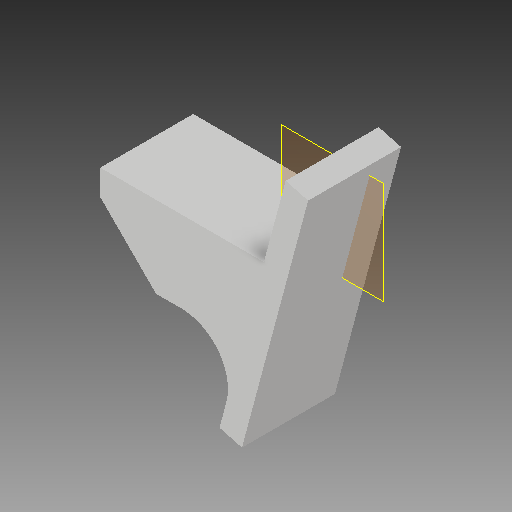
# Autodesk Inventor part: Stand_Back
Saved by Autodesk Inventor 2018 (Build 220112000, 112)
## iProperties
Created: 2018-02-04
Part Number: Stand_Back
Material: Generic
Document SubType Name: Modeling
Designer: Mandus
Density: 1 g/cm^3
Appearance: Default
Author: Mandus
Autodesk Inventor part; units mm, degrees
ref_plane "YZ Plane" through (0, 0, 0) normal (1, 0, 0) x (0, 1, 0)
sketch "Sketch1" plane through (0, 0, 0) normal (0, 0, 1) x (1, 0, 0)
  line L0 (36, 0.51) -> (25.6472, -38.1271)
  line L1 (36, 0.51) -> (76, 0.51) construction
  line L2 (36, 0.51) -> (25.6472, -38.1271) construction
  line L3 (25.6472, -38.1271) -> (30.4769, -39.4212)
  line L4 (30.4769, -39.4212) -> (40.8296, -0.7841)
  line L5 (40.8296, -0.7841) -> (36, 0.51)
  line L6 (36, 0.51) -> (40.8296, -0.7841)
  line L7 (40.8296, -0.7841) -> (44.7119, 13.7048)
  line L8 (44.7119, 13.7048) -> (39.8823, 14.9989)
  line L9 (39.8823, 14.9989) -> (36, 0.51)
  arc A0 (36, -1.5) -> (26, 8.5) centre (26, -1.5) ccw construction
  line L10 (39.0787, 12) -> (34.0787, 12)
  line L11 (34.0787, 12) -> (34.0787, 9)
  line L12 (34.0787, 9) -> (38.2749, 9)
  line L13 (14, -12.5) -> (26, -12.5) construction
  line L14 (0, -20) -> (30.5044, -20)
  line L15 (30.5044, -20) -> (35.8634, 0)
  line L16 (35.1935, -2.5) -> (0, -2.5)
  line L17 (35.1935, -2.5) -> (30.5044, -20)
  line L18 (0, -20) -> (0, -2.5)
  line L19 (-41.5, -2.5) -> (36, -2.5) construction
  line L20 (30.5044, -20) -> (35.1935, -2.5) construction
  point P0 (0, 0)
  point P1 (17.5967, -2.5)
  dimension "d0" = 40
  dimension "d1" = 105
  dimension "d2" = 5
  dimension "d3" = 15
  dimension "d5" = 5
  dimension "d6" = 3
  dimension "d7" = 11.49
  dimension "d20" = 17.5
  dimension "d21" = 35.1935
  dimension "d22" = 30.5044
  constraints: 42 end point, 5 point on line, 4 collinear, 4 horizontal, 4 parallel, 3 perpendicular, 3 vertical, 1 equal length, 1 horizontal alignment, 1 midpoint, 4 other
  measures "d0" distance of L0.start L0.end
  measures "d1" angle of L0 L1
  measures "d2" distance of L3.end L0.end
  measures "d3" distance of L7.end L4.end
  measures "d5" distance of L10.start L10.end
  measures "d6" distance of L10.end L11.end
  measures "d7" distance from line of L1 L10.end
  measures "d20" distance of L14.start L16.end
  measures "d21" distance of L16.start L16.end
  measures "d22" distance of L14.start L14.end
ref_plane "Work Plane1" through (0, 0, -20) normal (0, 0, -1) x (0, 1, 0)
extrude "Extrusion1" add sketch "Sketch1" against normal up to surface (20 mm away) contours L5 L4 L3 L0 | L9 L8 L7 L5 | L0 L14 L18 L16
ref_plane "Work Plane6" through (36, 0, -14) normal (0, 0, 1) x (1, 0, 0)
ref_plane "Work Plane3" through (0, 0.51, -6) normal (0, 0, -1) x (0, 1, 0)
fillet "Fillet2" radius 10 1 edges at (30.5044, -20, -10)
chamfer "Chamfer1" distance 12 angle 45 1 edges at (0, -20, -10)
body "Solid1"
